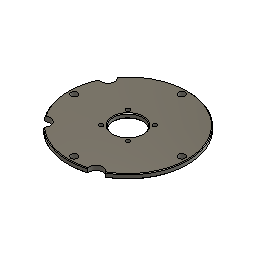
Motor_mount_base (Autodesk Fusion 360 design; units mm, degrees)
part number: 2025-04-19-22-32-25-468
Autodesk Fusion 360 part; units mm, degrees
sketch "Sketch1" plane through (0, 0, 0) normal (0, 1, 0) x (1, 0, 0)
  circle A0 centre (0, 0) radius 44.45
  circle A1 centre (-40, 0) radius 2.5
  circle A2 centre (0, -40) radius 2.5
  circle A3 centre (40, 0) radius 2.5
  circle A4 centre (0, 40) radius 2.5
  circle A5 centre (0, 0) radius 11
  line L0 (0, 0) -> (57.0088, 0) construction
  circle A6 centre (10, 10) radius 1.5
  circle A7 centre (-10, 10) radius 1.5
  circle A8 centre (-10, -10) radius 1.5
  circle A9 centre (10, -10) radius 1.5
  circle A10 centre (-33.6616, -29.0293) radius 5
  circle A11 centre (17.2065, -40.9846) radius 5
  circle A12 centre (-38.0105, 23.0436) radius 5
  dimension "d1" = 88.9
  dimension "d3" = 5
  dimension "d6" = 360
  dimension "d7" = 22
  dimension "d9" = 3
  dimension "d10" = 10
  dimension "d12" = 360
  dimension "d18" = 10
  dimension "d20" = 360
  constraint coincident A0.centre A5.centre
  constraint horizontal L0
  constraint coincident A0 A10.centre
  measures "d1" diameter of A0
  measures "d3" diameter of A1
  measures "d7" diameter of A5
  measures "d9" diameter of A6
  measures "d10" horizontal distance of A0.centre A6.centre
  measures "d18" diameter of A10
extrude "Extrude1" add sketch "Sketch1" along normal blind 3.5 contours A0 A10 A11 A12
chamfer "Chamfer1" distance 0.5 angle 45 1 edges at (-10.2556, 3.5, -3.9778)
chamfer "Chamfer2" distance 0.5 angle 45 1 edges at (-10.2556, 0, -3.9778)
chamfer "Chamfer3" distance 1 angle 45 4 edges at (8.6015, 0, 9.4576) (8.6015, 0, -10.5424) (-11.3985, 0, -10.5424) (-11.3985, 0, 9.4576)
chamfer "Chamfer4" distance 0.5 angle 45 6 edges at (33.6616, 3.5, -29.0293) (33.6616, 0, -29.0293) (-10.1698, 0, 43.271) (-10.1698, 3.5, 43.271) (-44.2958, 3.5, 3.6994) (-44.2958, 0, 3.6994)
